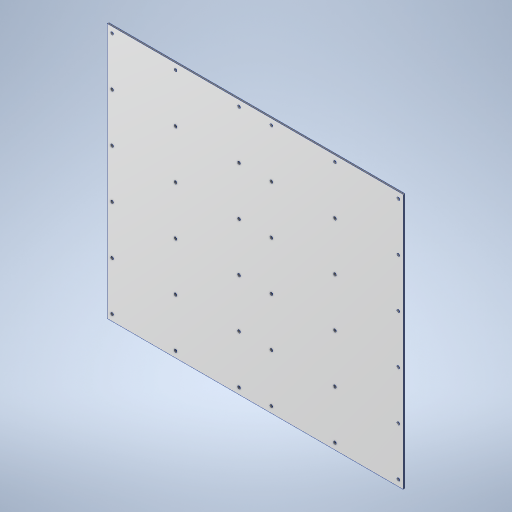
# Autodesk Inventor part: Rear Internal Side Panel R2
Saved by Autodesk Inventor 2024 (Build 280153000, 153)
## iProperties
Created: 2024-09-28
Part Number: Rear Internal Side Panel R2
Material: Generic
Document SubType Name: Modeling
Designer: Ishaan
Density: 1 g/cm^3
Appearance: Default
Author: Ishaan
Autodesk Inventor part; units mm, degrees
note: some values were not read from the file. Chosen so that the rebuilt part matches the saved one: hole positions of "Sketch Driven Pattern1".
ref_plane "YZ Plane" through (0, 0, 0) normal (1, 0, 0) x (0, 1, 0)
ref_plane "XZ Plane" through (0, 0, 0) normal (0, 1, 0) x (-1, 0, 0)
ref_plane "XY Plane" through (0, 0, 0) normal (0, 0, 1) x (1, 0, 0)
sketch "Sketch1" plane through (0, 0, 0) normal (0, 0, 1) x (1, 0, 0)
  line L0 (274, -236.5) -> (-274, -236.5)
  line L1 (-274, -236.5) -> (-274, 236.5)
  line L2 (-274, 236.5) -> (274, 236.5)
  line L3 (274, 236.5) -> (274, -236.5)
  line L4 (274, -236.5) -> (-274, 236.5) construction
  line L5 (-274, -236.5) -> (274, 236.5) construction
  point P0 (0, 0)
  dimension "d0" = 548
  dimension "d1" = 473
  constraints: 12 end point, 2 midpoint, 2 parallel, 1 horizontal, 1 perpendicular
  measures "d0" distance of L1.end L2.end
  measures "d1" distance of L0.end L1.end
extrude "Extrusion1" add sketch "Sketch1" along normal mid plane 3
extrude "Extrusion2" cut sketch "Sketch1" along normal mid plane 2.9
extrude "Extrusion3" add sketch "Sketch1" along normal mid plane 2.9 separate body
sketch "Sketch6" plane through (0, 0, 1.5) normal (0, 0, 1) x (1, 0, 0)
  line L0 (30, -225) -> (-30, -225) construction
  line L1 (-30, -225) -> (-30, 225) construction
  line L2 (-30, 225) -> (30, 225) construction
  line L3 (30, 225) -> (30, -225) construction
  line L4 (30, -225) -> (-30, 225) construction
  line L5 (-30, -225) -> (30, 225) construction
  line L6 (265, -225) -> (-265, -225) construction
  line L7 (-265, -225) -> (-265, 225) construction
  line L8 (-265, 225) -> (265, 225) construction
  line L9 (265, 225) -> (265, -225) construction
  line L10 (265, -225) -> (-265, 225) construction
  line L11 (-265, -225) -> (265, 225) construction
  point P0 (0, 0)
  point P1 (-265, 135)
  point P2 (-265, 45)
  point P3 (-265, -45)
  point P4 (-265, -135)
  dimension "d47" = 60
  dimension "d48" = 450
  dimension "d49" = 530
  dimension "d52" = 90
  constraints: 24 end point, 4 midpoint, 4 parallel, 2 coincident, 2 horizontal, 2 perpendicular, 1 collinear, 1 vertical, 5 other
  measures "d47" distance of L1.end L2.end
  measures "d48" distance of L2.end L0.start
  measures "d49" distance of L7.end L8.end
  measures "d52" distance of point (-265, 225) point (-265, 135)
hole "Hole4" at (-265, 225, 1.5) at (-265, 135, 1.5) at (-265, 45, 1.5) at (-265, -45, 1.5) at (-265, -135, 1.5) at (-265, -225, 1.5) direction (0, 0, -1) diameter 5.3 end through all bodies 1 2
sketch "Sketch8" plane through (0, 0, 1.5) normal (0, 0, 1) x (1, 0, 0)
  circle A0 centre (-265, 225) radius 2.65 projected
  point P0 (0, 0)
  point P1 (-147.5, 225)
  point P2 (-30, 225)
  point P3 (30, 225)
  point P4 (147.5, 225)
  point P5 (265, 225)
  dimension "d64" = 265
  dimension "d65" = 265
  dimension "d66" = 30
  dimension "d67" = 30
  dimension "d69" = 147.5
  dimension "d70" = 147.5
  constraints: 5 horizontal alignment, 1 coincident
  measures "d64" horizontal distance of point (-265, 225) point (0, 0)
  measures "d65" horizontal distance of point (265, 225) point (0, 0)
  measures "d66" horizontal distance of point (0, 0) point (-30, 225)
  measures "d67" horizontal distance of point (30, 225) point (0, 0)
  measures "d69" horizontal distance of point (0, 0) point (-147.5, 225)
  measures "d70" horizontal distance of point (147.5, 225) point (0, 0)
pattern_sketch "Sketch Driven Pattern1" of "Hole4" from (-265, 225, 1.5) bodies 1 2 copies at (-147.5, 225, 1.5) at (-30, 225, 1.5) at (30, 225, 1.5) at (147.5, 225, 1.5) at (265, 225, 1.5)
equation "\"d65\" = d64"
equation "\"d67\" = d66"
equation "\"d70\" = d69"
